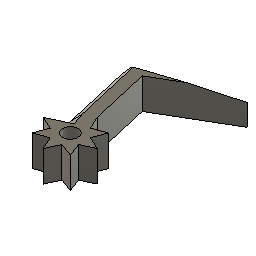
claw_part_right (Autodesk Fusion 360 design; units mm, degrees)
Autodesk Fusion 360 part; units mm, degrees
sketch "Sketch1" plane through (0, 0, 0) normal (0, 1, 0) x (1, 0, 0)
  line L0 (-7, 31.5) -> (-7, 0) construction
  line L1 (-35.9586, 21.9692) -> (-30.3122, -2.5628)
  line L2 (-7, 31.5) -> (-35.9586, 21.9692)
  line L3 (-22.2116, -4.1306) -> (-17.9378, -2.5628)
  line L4 (-27.5018, 14.6711) -> (-28.4889, 18.96)
  line L5 (-26.0384, -4.1306) -> (-24.125, 0)
  line L6 (-30.3122, -2.5628) -> (-24.125, 0)
  line L7 (-24.125, 0) -> (-17.9378, -2.5628)
  line L8 (-7, 31.5) -> (-14, -20.9929)
  line L9 (-7, 31.5) -> (-34.239, 31.5)
  circle A0 centre (-24.125, -8.75) radius 5
  line L10 (-24.125, 0) -> (-27.5018, 14.6711)
  circle A1 centre (-24.125, -8.75) radius 2.5
  line L11 (-30.3122, -14.9372) -> (-32.875, -8.75)
  line L12 (-28.7444, -10.6634) -> (-32.875, -8.75)
  line L13 (-17.9378, -2.5628) -> (-15.375, -8.75)
  line L14 (-24.125, -17.5) -> (-26.0384, -13.3694)
  line L15 (-43.7102, -20.9929) -> (-14, -20.9929)
  line L16 (-19.5056, -10.6634) -> (-17.9378, -14.9372)
  line L17 (-17.9378, -14.9372) -> (-24.125, -17.5)
  line L18 (-15.375, -8.75) -> (-17.9378, -14.9372)
  line L19 (-32.875, -8.75) -> (-28.7444, -6.8366)
  line L20 (-26.0384, -13.3694) -> (-30.3122, -14.9372)
  line L21 (-19.5056, -6.8366) -> (-15.375, -8.75)
  line L22 (-22.2116, -13.3694) -> (-24.125, -17.5)
  line L23 (-17.9378, -14.9372) -> (-22.2116, -13.3694)
  line L24 (-34.239, 31.5) -> (-43.7102, -20.9929)
  line L25 (-32.875, -8.75) -> (-30.3122, -2.5628)
  line L26 (-24.125, -17.5) -> (-30.3122, -14.9372)
  line L27 (-17.9378, -2.5628) -> (-19.5056, -6.8366)
  line L28 (-15.375, -8.75) -> (-19.5056, -10.6634)
  line L29 (-30.3122, -14.9372) -> (-28.7444, -10.6634)
  line L30 (-24.125, 0) -> (-22.2116, -4.1306)
  line L31 (-7, 31.5) -> (-28.4889, 18.96)
  line L32 (-29.1989, 4.3652) -> (-29.1875, 4.3554)
  line L33 (-30.3122, -2.5628) -> (-26.0384, -4.1306)
  line L34 (-21.0314, -1.2814) -> (-24.125, -8.75) construction
  line L35 (-28.7444, -6.8366) -> (-30.3122, -2.5628)
  point P0 (-24.125, -8.75)
  point P1 (-14, 0)
  point P2 (-14, 0)
  point P3 (-14, 0)
  point P4 (-7, 0)
  constraint symmetric origin L0 P3
  constraint symmetric L2.start L0 L8.start
  constraint symmetric P4 L0 L0.end
extrude "Extrude1" add sketch "Sketch1" along normal blind 10 contours L1 L2 L4 L6 L10 L31 | L5 L6 L33 | A0 L33 L35 | L5 A0 L30 | A0 L12 L19 | A0 | L3 A0 L27 | A0 L20 L29 | A0 L21 L28 | A0 L14 L22 | A0 L16 L23
chamfer "Chamfer3" distance 3 angle 45 1 edges at (-35.9586, 5, -21.9692)
chamfer "Chamfer4" distance 3 angle 45 1 edges at (-20.0545, 10, -27.2035)
chamfer "Chamfer5" distance 3 angle 45 2 edges at (-32.7975, 10, -8.2352) (-29.5283, 10, 4.6997)
